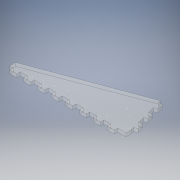
# Autodesk Inventor part: phone_holder_slider_side
Saved by Autodesk Inventor 2019 (Build 230136000, 136)
## iProperties
Created: 2019-02-17
Part Number: phone_holder_slider_side
Material: Acrylic, Clear
Document SubType Name: Modeling
Designer: suchanek
Density: 1.19 g/cm^3
Appearance: Transparent - Clear
Author: suchanek
Autodesk Inventor part; units mm, degrees
ref_plane "YZ Plane" through (0, 0, 0) normal (1, 0, 0) x (0, 1, 0)
ref_plane "XZ Plane" through (0, 0, 0) normal (0, 1, 0) x (-1, 0, 0)
ref_plane "XY Plane" through (0, 0, 0) normal (0, 0, 1) x (1, 0, 0)
sketch "Sketch2" plane through (0, 0, 0) normal (0, 1, 0) x (-1, 0, 0)
  line L0 (-100, 5) -> (100, 5)
  line L1 (100, 5) -> (100, -5)
  line L2 (100, -5) -> (-100, -5)
  line L3 (-100, -5) -> (-100, 5)
  line L4 (-100, 5) -> (100, -5) construction
  line L5 (100, 5) -> (-100, -5) construction
  line L6 (94, 11) -> (82, 11)
  line L7 (82, 11) -> (82, 5)
  line L8 (82, 5) -> (94, 5)
  line L9 (94, 5) -> (94, 11)
  line L10 (70, 11) -> (58, 11)
  line L11 (70, 5) -> (70, 11)
  line L12 (58, 11) -> (58, 5)
  line L13 (58, 5) -> (70, 5)
  line L14 (46, 11) -> (34, 11)
  line L15 (46, 5) -> (46, 11)
  line L16 (34, 11) -> (34, 5)
  line L17 (34, 5) -> (46, 5)
  line L18 (22, 11) -> (10, 11)
  line L19 (22, 5) -> (22, 11)
  line L20 (10, 11) -> (10, 5)
  line L21 (10, 5) -> (22, 5)
  line L22 (-2, 11) -> (-14, 11)
  line L23 (-2, 5) -> (-2, 11)
  line L24 (-14, 11) -> (-14, 5)
  line L25 (-14, 5) -> (-2, 5)
  line L26 (-26, 11) -> (-38, 11)
  line L27 (-26, 5) -> (-26, 11)
  line L28 (-38, 11) -> (-38, 5)
  line L29 (-38, 5) -> (-26, 5)
  line L30 (-50, 11) -> (-62, 11)
  line L31 (-50, 5) -> (-50, 11)
  line L32 (-62, 11) -> (-62, 5)
  line L33 (-62, 5) -> (-50, 5)
  line L34 (-74, 11) -> (-86, 11)
  line L35 (-74, 5) -> (-74, 11)
  line L36 (-86, 11) -> (-86, 5)
  line L37 (-86, 5) -> (-74, 5)
  line L38 (-100, -5) -> (-81.8827, -72.6148)
  line L39 (-100, -5) -> (-30, -5) construction
  line L40 (-81.8827, -72.6148) -> (100, -5)
  line L41 (-83.1768, -67.7852) -> (-86.2826, -56.1941)
  line L42 (-86.2826, -56.1941) -> (-92.0781, -57.747)
  line L43 (-92.0781, -57.747) -> (-88.9723, -69.3381)
  line L44 (-88.9723, -69.3381) -> (-83.1768, -67.7852)
  line L45 (-89.3884, -44.603) -> (-92.4942, -33.0118)
  line L46 (-95.184, -46.1559) -> (-89.3884, -44.603)
  line L47 (-98.2898, -34.5648) -> (-95.184, -46.1559)
  line L48 (-92.4942, -33.0118) -> (-98.2898, -34.5648)
  line L49 (-95.6001, -21.4207) -> (-98.7059, -9.8296)
  line L50 (-101.3956, -22.9737) -> (-95.6001, -21.4207)
  line L51 (-104.5015, -11.3825) -> (-101.3956, -22.9737)
  line L52 (-98.7059, -9.8296) -> (-104.5015, -11.3825)
  point P0 (0, 0)
  dimension "d9" = 10
  dimension "d10" = 200
  dimension "d19" = 12
  dimension "d20" = 6
  dimension "d21" = 6
  dimension "d35" = 24
  dimension "d40" = 70
  dimension "d41" = 75
  dimension "d42" = 6
  dimension "d45" = 24
  dimension "d50" = 5
  dimension "d51" = 12
  constraints: 106 end point, 6 parallel, 4 horizontal, 3 perpendicular, 2 midpoint, 2 point on line, 1 collinear, 1 equal length, 73 other
  measures "d9" distance of L0.end L1.end
  measures "d10" distance of L1.end L2.end
  measures "d19" distance of L8.end L7.end
  measures "d20" distance of L7.end L6.end
  measures "d21" distance between parallel lines of L1 L9
  measures "d35" distance of L6.start L10.start
  measures "d40" distance of L2.end L38.end
  measures "d41" angle of L38 L39
  measures "d42" distance of L42.end L41.end
  measures "d45" distance of L41.end L45.end
  measures "d50" distance from line of L38.end L44
  measures "d51" distance of L42.end L43.end
extrude "Extrusion2" add sketch "Sketch2" along normal blind 6
body "Solid2"
